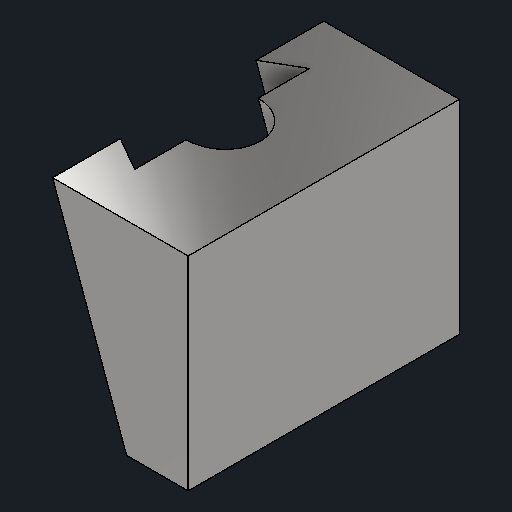
# Autodesk Inventor part: Part1
Saved by Autodesk Inventor 2026.2 (Build 302298000, 298)
## iProperties
Created: 2026-09-23
Part Number: Part1
Material: Steel, Alloy
Document SubType Name: Modeling
Designer: JoshuaEah
Density: 7.73 g/cm^3
Appearance: Semi-Polished
Author: JoshuaEah
Autodesk Inventor part; units mm, degrees
ref_plane "YZ Plane" through (0, 0, 0) normal (1, 0, 0) x (0, 1, 0)
ref_plane "XZ Plane" through (0, 0, 0) normal (0, 1, 0) x (-1, 0, 0)
sketch "Sketch1" plane through (0, 0, 0) normal (0, 1, 0) x (-1, 0, 0)
  line L0 (0, 0) -> (-12.7, 0)
  line L1 (-12.7, 0) -> (-12.7, -25.4)
  line L2 (-12.7, -25.4) -> (0, -25.4)
  line L3 (0, -25.4) -> (0, 0)
  line L4 (0, -12.7) -> (-12.7, -12.7) construction
  line L5 (-3.175, -25.4) -> (-3.175, 0)
  line L6 (-3.175, -20.8831) -> (0, -19.05)
  line L7 (-3.175, -4.5169) -> (0, -6.35)
  point P0 (-3.175, -12.7)
  point P1 (0, -6.35)
  dimension "d0" = 12.7
  dimension "d7" = 25.4
  dimension "d34" = 3.175
  dimension "d35" = 60
  dimension "d36" = 12.7
  constraints: 16 end point, 4 point on line, 3 midpoint, 2 parallel, 2 perpendicular, 2 symmetric about line, 1 coincident, 1 horizontal
  measures "d0" distance of L2.end L1.end
  measures "d7" distance of L2.end L0.start
  measures "d34" distance between parallel lines of L3 L5
  measures "d35" angle of L3 L6
  measures "d36" diameter of L6.end L4
extrude "Extrusion2" add sketch "Sketch1" against normal blind 19.05
sketch "Sketch6" plane through (0, 0, 0) normal (0, 0, 1) x (-1, 0, 0)
  line L0 (0, 0) -> (-12.7, 0) projected
  line L1 (-12.7, 0) -> (-12.7, 19.05) projected
  line L2 (-12.7, 19.05) -> (0, 19.05) projected
  line L3 (0, 0) -> (0, 19.05) projected
  line L4 (0, 0) -> (-6.9336, 19.05)
  dimension "d41" = 70
  constraints: 2 end point, 1 point on line
  measures "d41" angle of L2 L4
sweep "Sweep2" cut profiles "Sketch1" path "Sketch6" path curves L4 contours L3 L6 L5 L7
ref_plane "Work Plane5" through (3.175, 0, -25.4) normal (-0.3420201, 0.9396926, 0) x (0, 0, 1)
ref_plane "Work Plane4" through (0, 0, -25.4) normal (0.9396926, 0.3420201, 0) x (0, 0, 1)
sketch "Sketch7" plane through (3.175, 0, -25.4) normal (-0.3420201, 0.9396926, 0) x (0, 0, 1)
  point P0 (12.7, 0)
hole "Hole3" at (3.175, 0, -12.7) direction (0.3420201, -0.9396926, 0) diameter 6.7564 depth 12.7 tip angle 118
split "Split2" plane through (0, 0, -25.4) removes the side toward (-0.9396926, -0.3420201, 0)
equation "\"d41\" = slopeAngle"
equation "\"slopeAngle\" = 70deg"
equation "\"d44\" = -slopeAngle"
body "Solid3"
